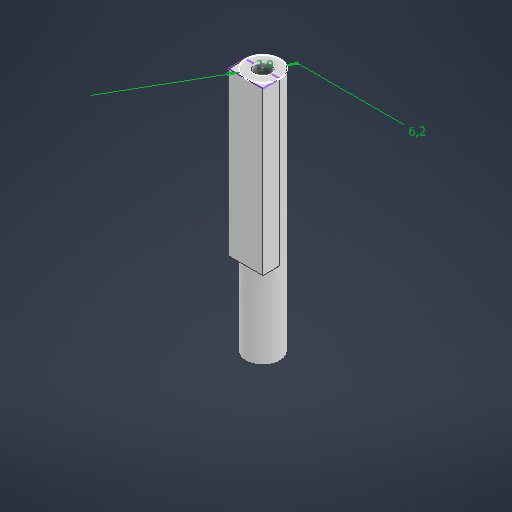
# Autodesk Inventor part: spojka v2
Saved by Autodesk Inventor 2026 (Build 300175000, 175)
## iProperties
Created: 2025-07-12
Part Number: spojka v2
Material: Všeobecné
Document SubType Name: Modeling
Designer: vadim
Density: 1 g/cm^3
Appearance: Výchozí
Author: vadim
Autodesk Inventor part; units mm, degrees
ref_plane "YZ Plane" through (0, 0, 0) normal (1, 0, 0) x (0, 1, 0)
ref_plane "XZ Plane" through (0, 0, 0) normal (0, 1, 0) x (-1, 0, 0)
ref_plane "XY Plane" through (0, 0, 0) normal (0, 0, 1) x (1, 0, 0)
sketch "Náčrt1" plane through (0, 0, 0) normal (0, 1, 0) x (-1, 0, 0)
  circle A0 centre (0, 0) radius 3.1
  circle A1 centre (0, 0) radius 1.45
  line L0 (3.1, 0) -> (-3.1, 0)
  line L1 (-3.1, 0) -> (-3.1, 3.1)
  line L2 (-3.1, 3.1) -> (3.1, 3.1)
  line L3 (3.1, 3.1) -> (3.1, 0)
  point P0 (0, 3.1)
  dimension "d0" = 6.2
  dimension "d1" = 2.9
  constraints: 8 end point, 2 coincident, 2 parallel, 1 centre point, 1 horizontal, 1 perpendicular, 3 other
  measures "d1" diameter of A1
extrude "Vysunutí1" add sketch "Náčrt1" against normal blind 44.2 contours L0 A1 A0 | A0 L0 A1 | L0 A1 | A1 L0
extrude "Vysunutí2" add sketch "Náčrt1" against normal blind 29.3 contours L1 L2 A0 | A0 L2 L3
sketch "Náčrt2" plane through (0, 0, 0) normal (0, 1, 0) x (1, 0, 0)
  circle A0 centre (0, 0) radius 3.1 projected
  point P0 (-3.1, 0)
  point P1 (3.1, 0)
  constraints: 1 coincident
hole "Díra1" at (0, 0, 0) direction (0, -1, 0) diameter 2.9 depth 10
sketch "Náčrt3" plane through (0, -44.2, 0) normal (0, -1, 0) x (1, 0, 0)
  circle A0 centre (0, 0) radius 3.1 projected
  point P0 (3.1, 0)
  point P1 (-3.1, 0)
  constraints: 1 coincident
hole "Díra2" at (0, -44.2, 0) direction (0, 1, 0) diameter 2.85 depth 4.5
